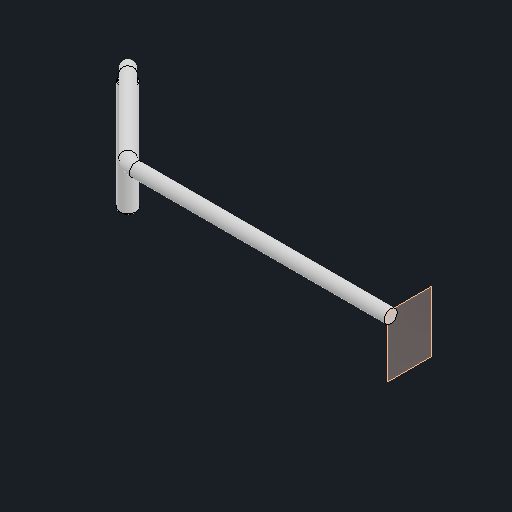
# Autodesk Inventor part: 5th Wheel Hitch Part 4
Saved by Autodesk Inventor 2025.1 (Build 291241000, 241)
## iProperties
Created: 2026-02-23
Part Number: 5th Wheel Hitch Part 4
Material: Generic
Document SubType Name: Modeling
Designer: Desktop -24
Density: 1 g/cm^3
Appearance: Default
Author: Desktop -24
Autodesk Inventor part; units mm, degrees
ref_plane "XZ Plane" through (0, 0, 0) normal (0, 1, 0) x (-1, 0, 0)
ref_plane "XY Plane" through (0, 0, 0) normal (0, 0, 1) x (1, 0, 0)
ref_plane "Work Plane1" through (508, 0, 0) normal (1, 0, 0) x (0, 1, 0)
sketch "Sketch13" plane through (508, 0, 0) normal (1, 0, 0) x (0, 1, 0)
  circle A0 centre (0, 0) radius 12.7
  point P0 (0, 0)
  dimension "d79" = 25.4
  constraints: 1 centre point, 1 coincident
  measures "d79" diameter of A0
sketch3d "3D Sketch1"
  line L0 (508, 0, 0) -> (15.7815, 0, 0)
  arc A0 (15.7815, 0, 0) -> (-11.1592, 0.0018, -11.1592) centre (15.7815, 0.0061, -38.1) ccw
  line L1 (-11.1592, 0.0018, -11.1592) -> (-152.6613, 0.0245, -152.6613)
  arc A1 (-152.6613, 0.0245, -152.6613) -> (-179.6051, -38.0755, -179.6051) centre (-152.6644, -38.0755, -152.6644) ccw
  line L2 (-179.6051, -38.0755, -179.6051) -> (-179.6051, -253.9712, -179.6051)
  dimension "d73" = 508
  dimension "d74" = 135
  dimension "d75" = 254
  dimension "d76" = 254
  dimension "d77" = 38.1
  dimension "d78" = 38.1
sweep "Sweep1" add profiles "Sketch13" path "3D Sketch1"
sketch "Sketch14" plane through (-179.6051, -253.9712, -179.6051) normal (0, -1, 0) x (1, 0, 0)
  circle A0 centre (0, 0.1847) radius 15.875
  point P0 (179.6051, 179.6051)
  dimension "d82" = 31.75
  constraints: 1 centre point
  measures "d82" diameter of A0
extrude "Extrusion1" add sketch "Sketch14" against normal blind 215.9
fillet "Fillet1" radius 3.175 1 edges at (-195.4801, -253.9712, -179.4205)
fillet "Fillet2" radius 1.5875 1 edges at (-195.4801, -38.0712, -179.4205)
equation "\"d78\" = d77"
equation "\"BendRadius\" = Thickness"
equation "\"BendReliefWidth\" = Thickness"
equation "\"BendReliefDepth\" = 0.5 * Thickness"
equation "\"CornerReliefSize\" = 4 * Thickness"
equation "\"MinimumRemnant\" = 2 * Thickness"
equation "\"TransitionRadius\" = BendRadius"
equation "\"JacobiRadiusSize\" = BendRadius"
equation "\"GapSize\" = Thickness"
equation "\"Thickness\" = 9.525"
body "Solid2"
